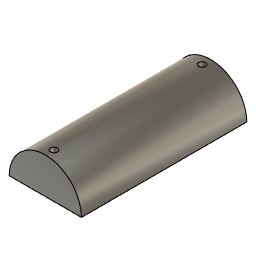
Stepper Fixture v1 (Autodesk Fusion 360 design; units mm, degrees)
Autodesk Fusion 360 part; units mm, degrees
sketch "Sketch1" plane through (0, 0, 0) normal (0, 1, 0) x (1, 0, 0)
  line L0 (0, 0) -> (42, 0)
  arc A0 (0, 0) -> (42, 0) centre (21, 0) ccw
  dimension "d1" = 42
  constraint coincident L0.start A0.start
  constraint horizontal L0
  measures "d1" distance of L0.start L0.end
extrude "Extrude1" add sketch "Sketch1" along normal blind 96.2
sketch "Sketch2" plane through (0, 0, 0) normal (0, 0, -1) x (1, 0, 0)
  line L0 (42, 0) -> (0, 0)
  line L1 (0, 0) -> (0, -96.2)
  line L2 (0, -96.2) -> (42, -96.2)
  line L3 (42, -96.2) -> (42, 0)
  circle A0 centre (21, -5) radius 2
  circle A1 centre (21, -91.2) radius 2
  dimension "d6" = 4
  dimension "d7" = 4
  dimension "d10" = 5
  dimension "d11" = 5
  measures "d6" diameter of A0
  measures "d7" diameter of A1
  measures "d10" distance of L0 A0.centre
  measures "d11" distance of L2 A1.centre
extrude "Extrude2" cut sketch "Sketch2" against normal blind 26.592 contours A0 | A1
